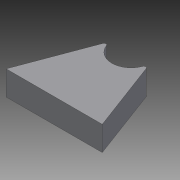
# Autodesk Inventor part: Air2D_Shaft_Brace
Saved by Autodesk Inventor 2014 (Build 180170000, 170)
## iProperties
Created: 2014-09-30
Part Number: Air2D_Shaft_Brace
Material: Generic
Document SubType Name: Modeling
Designer: ThatOtherGuy
Density: 1 g/cm^3
Appearance: Default
Author: ThatOtherGuy
Autodesk Inventor part; units mm, degrees
ref_plane "YZ Plane" through (0, 0, 0) normal (1, 0, 0) x (0, 1, 0)
ref_plane "XZ Plane" through (0, 0, 0) normal (0, 1, 0) x (-1, 0, 0)
ref_plane "XY Plane" through (0, 0, 0) normal (0, 0, 1) x (1, 0, 0)
sketch "Sketch1" plane through (0, 0, 0) normal (0, 0, 1) x (1, 0, 0)
  line L0 (0, 0) -> (25, 0)
  arc A0 (7.8015, 18.2899) -> (17.1985, 18.2899) centre (12.5, 20) ccw
  line L1 (18.1364, 18.2945) -> (25, 0)
  line L2 (6.8636, 18.2945) -> (0, 0)
  arc A1 (7.8015, 18.2899) -> (6.8636, 18.2945) centre (7.3317, 18.1189) ccw
  arc A2 (18.1364, 18.2945) -> (17.1985, 18.2899) centre (17.6683, 18.1189) ccw
  dimension "d0" = 5
  dimension "d1" = 20
  dimension "d2" = 25
  dimension "d4" = 20
  dimension "d9" = 0.5
  constraints: 6 end point, 6 point on circle, 4 tangent, 3 centre point, 1 equal length, 1 equal radius, 1 horizontal, 1 horizontal alignment
  measures "d0" radius of A0
  measures "d1" distance from line of L0 A0.centre
  measures "d2" distance of L0.start L0.end
  measures "d9" radius of A2
extrude "Extrusion1" add sketch "Sketch1" along normal blind 3.175
equation "\"d5\" = THICKA"
equation "\"THICKA\" = 3.175"
equation "\"THICKB\" = 6.731"
equation "\"THICKC\" = 12.7"
equation "\"MAGDIA\" = 9.5"
equation "\"BALLDIA\" = 12"
body "Solid1"
